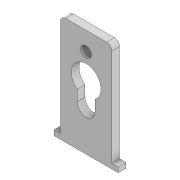
# Autodesk Inventor part: vtail_slide_in
Saved by Autodesk Inventor 2022 (Build 260153000, 153)
## iProperties
Created: 2022-05-19
Part Number: vtail_slide_in
Material: Generic
Document SubType Name: Modeling
Designer: Thomas
Density: 1 g/cm^3
Appearance: Default
Author: Thomas
Autodesk Inventor part; units mm, degrees
ref_plane "YZ Plane" through (0, 0, 0) normal (1, 0, 0) x (0, 1, 0)
ref_plane "XZ Plane" through (0, 0, 0) normal (0, 1, 0) x (-1, 0, 0)
ref_plane "XY Plane" through (0, 0, 0) normal (0, 0, 1) x (1, 0, 0)
sketch "Sketch1" plane through (0, 0, 0) normal (0, 0, 1) x (1, 0, 0)
  circle A0 centre (0, 0) radius 5.75
  line L0 (0, 0) -> (0, -8.8) construction
  line L1 (-3.45, 0) -> (-3.45, -8.8)
  line L2 (3.45, -8.8) -> (3.45, 0)
  arc A1 (3.45, 0) -> (-3.45, 0) centre (0, 0) ccw
  arc A2 (-3.45, -8.8) -> (3.45, -8.8) centre (0, -8.8) ccw
  line L3 (-10, 17) -> (10, 17)
  line L4 (10, 17) -> (10, -22.8)
  line L5 (10, -22.8) -> (-10, -22.8)
  line L6 (-10, -22.8) -> (-10, 17)
  circle A3 centre (0, 9.7) radius 2.1
  line L7 (-12.5, -22.8) -> (12.5, -22.8)
  line L8 (12.5, -22.8) -> (12.5, -24.8)
  line L9 (12.5, -24.8) -> (-12.5, -24.8)
  line L10 (-12.5, -24.8) -> (-12.5, -22.8)
  point P0 (0, -4.4)
  point P1 (-3.45, -4.6)
  point P2 (3.45, -4.6)
  dimension "d0" = 11.5
  dimension "d1" = 6.9
  dimension "d2" = 18
  dimension "d3" = 20
  dimension "d4" = 10
  dimension "d5" = 17
  dimension "d6" = 14
  dimension "d7" = 4.2
  dimension "d8" = 18.5
  dimension "d9" = 10
  dimension "d12" = 25
  dimension "d13" = 14
  dimension "d14" = 2.5
  dimension "d15" = 2
  constraints: 24 end point, 5 parallel, 4 centre point, 4 point on circle, 4 tangent, 2 horizontal, 2 perpendicular, 1 coincident, 1 midpoint, 1 vertical
  measures "d0" diameter of A0
  measures "d1" distance between parallel lines of L1 L2
  measures "d3" distance of L3.start L3.end
  measures "d4" distance from line of L6 point (0, 0)
  measures "d5" distance from line of point (0, 0) L3
  measures "d6" distance from line of L5 L0.end
  measures "d7" diameter of A3
  measures "d8" distance of L0.end A3.centre
  measures "d9" distance from line of L6 A3.centre
  measures "d12" distance of L8.end L9.end
  measures "d13" distance from line of L0.end L7
  measures "d14" distance between parallel lines of L4 L8
  measures "d15" distance from line of L4.end L9
extrude "Extrusion1" add sketch "Sketch1" along normal blind 3
fillet "Fillet1" radius 2 2 edges at (10, 17, 1.5) (-10, 17, 1.5)
equation "\"d4\" = 0.5 * d3"
equation "\"d9\" = d4"
equation "\"d14\" = -0.5 * d3 + 0.5 * d12"
body "Solid1"
